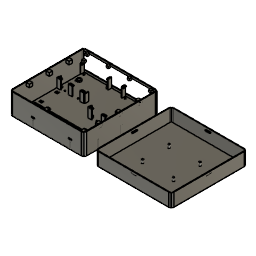
test slicing (Autodesk Fusion 360 design; units mm, degrees)
part number: 2026-06-28-20-30-48-696
Autodesk Fusion 360 part; units mm, degrees
sketch "Sketch1" plane through (0, 0, 0) normal (0, 0, 1) x (1, 0, 0)
  line L0 (140, 140) -> (-140, 140)
  line L1 (-140, 140) -> (-140, -140)
  line L2 (-140, -140) -> (140, -140)
  line L3 (140, -140) -> (140, 140)
extrude "Extrude1" add sketch "Sketch1" along normal blind 3 makes body 1
sketch "Sketch2" plane through (0, 0, 0) normal (0, 0, 1) x (1, 0, 0)
  line L0 (-137, 140) -> (-140, 140)
  line L1 (-140, 140) -> (-140, -140)
  line L2 (-140, -140) -> (-137, -140)
  line L3 (-137, -140) -> (-137, 140)
extrude "Extrude2" add sketch "Sketch2" along normal blind 77 from surface at 3 bodies 1
sketch "Sketch3" plane through (0, 0, 0) normal (0, 0, 1) x (1, 0, 0)
  line L0 (140, 140) -> (137, 140)
  line L1 (137, 140) -> (137, -140)
  line L2 (137, -140) -> (140, -140)
  line L3 (140, -140) -> (140, 140)
extrude "Extrude3" add sketch "Sketch3" along normal blind 77 from surface at 3 bodies 1
sketch "Sketch4" plane through (0, 0, 0) normal (0, 0, 1) x (1, 0, 0)
  line L0 (140, -137) -> (-140, -137)
  line L1 (-140, -137) -> (-140, -140)
  line L2 (-140, -140) -> (140, -140)
  line L3 (140, -140) -> (140, -137)
extrude "Extrude4" add sketch "Sketch4" along normal blind 77 from surface at 3 bodies 1
sketch "Sketch5" plane through (0, 0, 0) normal (0, 0, 1) x (1, 0, 0)
  line L0 (140, 140) -> (-140, 140)
  line L1 (-140, 140) -> (-140, 137)
  line L2 (-140, 137) -> (140, 137)
  line L3 (140, 137) -> (140, 140)
extrude "Extrude5" add sketch "Sketch5" along normal blind 8 from surface at 3 bodies 1
sketch "Sketch6" plane through (0, 0, 0) normal (0, 0, 1) x (1, 0, 0)
  line L0 (140, 140) -> (-140, 140)
  line L1 (-140, 140) -> (-140, 137)
  line L2 (-140, 137) -> (140, 137)
  line L3 (140, 137) -> (140, 140)
extrude "Extrude6" add sketch "Sketch6" along normal blind 8 from surface at 72 bodies 1
fillet "Fillet1" radius 10 4 edges at (-140, 140, 40) (-140, -140, 40) (140, -140, 40) (140, 140, 40) on bodies 1
sketch "Sketch7" plane through (0, 0, 0) normal (0, 0, 1) x (1, 0, 0)
  circle A0 centre (27, 128.5) radius 3.5
extrude "Extrude7" add sketch "Sketch7" along normal blind 3.5 from surface at 3 bodies 1
sketch "Sketch8" plane through (0, 0, 0) normal (0, 0, 1) x (1, 0, 0)
  circle A0 centre (27, 5.5) radius 3.5
extrude "Extrude8" add sketch "Sketch8" along normal blind 3.5 from surface at 3 bodies 1
sketch "Sketch9" plane through (0, 0, 0) normal (0, 0, 1) x (1, 0, 0)
  circle A0 centre (129, 128.5) radius 3.5
extrude "Extrude9" add sketch "Sketch9" along normal blind 3.5 from surface at 3 bodies 1
sketch "Sketch10" plane through (0, 0, 0) normal (0, 0, 1) x (1, 0, 0)
  circle A0 centre (129, 5.5) radius 3.5
extrude "Extrude10" add sketch "Sketch10" along normal blind 3.5 from surface at 3 bodies 1
sketch "Sketch11" plane through (0, 0, 0) normal (0, 0, 1) x (1, 0, 0)
  line L0 (34.5, -3) -> (20.5, -3)
  line L1 (20.5, -3) -> (20.5, -5.5)
  line L2 (20.5, -5.5) -> (34.5, -5.5)
  line L3 (34.5, -5.5) -> (34.5, -3)
extrude "Extrude11" add sketch "Sketch11" along normal blind 36.5 from surface at 3 bodies 1
sketch "Sketch12" plane through (0, 0, 0) normal (0, 0, 1) x (1, 0, 0)
  line L0 (34.5, 2.25) -> (20.5, 2.25)
  line L1 (20.5, 2.25) -> (20.5, -4.25)
  line L2 (20.5, -4.25) -> (34.5, -4.25)
  line L3 (34.5, -4.25) -> (34.5, 2.25)
extrude "Extrude12" add sketch "Sketch12" along normal blind 3 from surface at 35.5 bodies 1
sketch "Sketch13" plane through (0, 0, 0) normal (0, 0, 1) x (1, 0, 0)
  line L0 (85, -3) -> (71, -3)
  line L1 (71, -3) -> (71, -5.5)
  line L2 (71, -5.5) -> (85, -5.5)
  line L3 (85, -5.5) -> (85, -3)
extrude "Extrude13" add sketch "Sketch13" along normal blind 36.5 from surface at 3 bodies 1
sketch "Sketch14" plane through (0, 0, 0) normal (0, 0, 1) x (1, 0, 0)
  line L0 (85, 2.25) -> (71, 2.25)
  line L1 (71, 2.25) -> (71, -4.25)
  line L2 (71, -4.25) -> (85, -4.25)
  line L3 (85, -4.25) -> (85, 2.25)
extrude "Extrude14" add sketch "Sketch14" along normal blind 3 from surface at 35.5 bodies 1
sketch "Sketch15" plane through (0, 0, 0) normal (0, 0, 1) x (1, 0, 0)
  line L0 (135.5, -3) -> (121.5, -3)
  line L1 (121.5, -3) -> (121.5, -5.5)
  line L2 (121.5, -5.5) -> (135.5, -5.5)
  line L3 (135.5, -5.5) -> (135.5, -3)
extrude "Extrude15" add sketch "Sketch15" along normal blind 36.5 from surface at 3 bodies 1
sketch "Sketch16" plane through (0, 0, 0) normal (0, 0, 1) x (1, 0, 0)
  line L0 (135.5, 2.25) -> (121.5, 2.25)
  line L1 (121.5, 2.25) -> (121.5, -4.25)
  line L2 (121.5, -4.25) -> (135.5, -4.25)
  line L3 (135.5, -4.25) -> (135.5, 2.25)
extrude "Extrude16" add sketch "Sketch16" along normal blind 3 from surface at 35.5 bodies 1
sketch "Sketch17" plane through (0, 0, 0) normal (0, 0, 1) x (1, 0, 0)
  line L0 (20.5, 11) -> (18, 11)
  line L1 (18, 11) -> (18, -3)
  line L2 (18, -3) -> (20.5, -3)
  line L3 (20.5, -3) -> (20.5, 11)
extrude "Extrude17" add sketch "Sketch17" along normal blind 32.5 from surface at 3 bodies 1
sketch "Sketch18" plane through (0, 0, 0) normal (0, 0, 1) x (1, 0, 0)
  line L0 (20.5, 137) -> (18, 137)
  line L1 (18, 137) -> (18, 123)
  line L2 (18, 123) -> (20.5, 123)
  line L3 (20.5, 123) -> (20.5, 137)
extrude "Extrude18" add sketch "Sketch18" along normal blind 37.5 from surface at 3 bodies 1
sketch "Sketch19" plane through (0, 0, 0) normal (0, 0, 1) x (1, 0, 0)
  line L0 (24.5, 137) -> (18, 137)
  line L1 (18, 137) -> (18, 123)
  line L2 (18, 123) -> (24.5, 123)
  line L3 (24.5, 123) -> (24.5, 137)
extrude "Extrude19" add sketch "Sketch19" along normal blind 3 from surface at 35.5 bodies 1
sketch "Sketch20" plane through (0, 0, 0) normal (0, 0, 1) x (1, 0, 0)
  line L0 (51, 0.5) -> (48, 0.5)
  line L1 (48, 0.5) -> (48, -2.5)
  line L2 (48, -2.5) -> (51, -2.5)
  line L3 (51, -2.5) -> (51, 0.5)
extrude "Extrude20" add sketch "Sketch20" along normal blind 3 from surface at 3 bodies 1
sketch "Sketch21" plane through (0, 0, 0) normal (0, 0, 1) x (1, 0, 0)
  line L0 (138, 11) -> (135.5, 11)
  line L1 (135.5, 11) -> (135.5, -3)
  line L2 (135.5, -3) -> (138, -3)
  line L3 (138, -3) -> (138, 11)
extrude "Extrude21" add sketch "Sketch21" along normal blind 32.5 from surface at 3 bodies 1
sketch "Sketch22" plane through (0, 0, 0) normal (0, 0, 1) x (1, 0, 0)
  line L0 (138, 137) -> (135.5, 137)
  line L1 (135.5, 137) -> (135.5, 123)
  line L2 (135.5, 123) -> (138, 123)
  line L3 (138, 123) -> (138, 137)
extrude "Extrude22" add sketch "Sketch22" along normal blind 37.5 from surface at 3 bodies 1
sketch "Sketch23" plane through (0, 0, 0) normal (0, 0, 1) x (1, 0, 0)
  line L0 (138, 137) -> (131.5, 137)
  line L1 (131.5, 137) -> (131.5, 123)
  line L2 (131.5, 123) -> (138, 123)
  line L3 (138, 123) -> (138, 137)
extrude "Extrude23" add sketch "Sketch23" along normal blind 3 from surface at 35.5 bodies 1
sketch "Sketch24" plane through (0, 0, 0) normal (0, 0, 1) x (1, 0, 0)
  line L0 (108, 0.5) -> (105, 0.5)
  line L1 (105, 0.5) -> (105, -2.5)
  line L2 (105, -2.5) -> (108, -2.5)
  line L3 (108, -2.5) -> (108, 0.5)
extrude "Extrude24" add sketch "Sketch24" along normal blind 3 from surface at 3 bodies 1
sketch "Sketch25" plane through (0, 0, 0) normal (0, 0, 1) x (1, 0, 0)
  circle A0 centre (-129, 128.5) radius 3.5
extrude "Extrude25" add sketch "Sketch25" along normal blind 3.5 from surface at 3 bodies 1
sketch "Sketch26" plane through (0, 0, 0) normal (0, 0, 1) x (1, 0, 0)
  circle A0 centre (-129, 44.5) radius 3.5
extrude "Extrude26" add sketch "Sketch26" along normal blind 3.5 from surface at 3 bodies 1
sketch "Sketch27" plane through (0, 0, 0) normal (0, 0, 1) x (1, 0, 0)
  circle A0 centre (-41, 128.5) radius 3.5
extrude "Extrude27" add sketch "Sketch27" along normal blind 3.5 from surface at 3 bodies 1
sketch "Sketch28" plane through (0, 0, 0) normal (0, 0, 1) x (1, 0, 0)
  circle A0 centre (-41, 44.5) radius 3.5
extrude "Extrude28" add sketch "Sketch28" along normal blind 3.5 from surface at 3 bodies 1
sketch "Sketch29" plane through (0, 0, 0) normal (0, 0, 1) x (1, 0, 0)
  line L0 (-121.5, 36) -> (-135.5, 36)
  line L1 (-135.5, 36) -> (-135.5, 33.5)
  line L2 (-135.5, 33.5) -> (-121.5, 33.5)
  line L3 (-121.5, 33.5) -> (-121.5, 36)
extrude "Extrude29" add sketch "Sketch29" along normal blind 35.5 from surface at 3 bodies 1
sketch "Sketch30" plane through (0, 0, 0) normal (0, 0, 1) x (1, 0, 0)
  line L0 (-121.5, 41.25) -> (-135.5, 41.25)
  line L1 (-135.5, 41.25) -> (-135.5, 34.75)
  line L2 (-135.5, 34.75) -> (-121.5, 34.75)
  line L3 (-121.5, 34.75) -> (-121.5, 41.25)
extrude "Extrude30" add sketch "Sketch30" along normal blind 3 from surface at 34.5 bodies 1
sketch "Sketch31" plane through (0, 0, 0) normal (0, 0, 1) x (1, 0, 0)
  line L0 (-78, 36) -> (-92, 36)
  line L1 (-92, 36) -> (-92, 33.5)
  line L2 (-92, 33.5) -> (-78, 33.5)
  line L3 (-78, 33.5) -> (-78, 36)
extrude "Extrude31" add sketch "Sketch31" along normal blind 35.5 from surface at 3 bodies 1
sketch "Sketch32" plane through (0, 0, 0) normal (0, 0, 1) x (1, 0, 0)
  line L0 (-78, 41.25) -> (-92, 41.25)
  line L1 (-92, 41.25) -> (-92, 34.75)
  line L2 (-92, 34.75) -> (-78, 34.75)
  line L3 (-78, 34.75) -> (-78, 41.25)
extrude "Extrude32" add sketch "Sketch32" along normal blind 3 from surface at 34.5 bodies 1
sketch "Sketch33" plane through (0, 0, 0) normal (0, 0, 1) x (1, 0, 0)
  line L0 (-34.5, 36) -> (-48.5, 36)
  line L1 (-48.5, 36) -> (-48.5, 33.5)
  line L2 (-48.5, 33.5) -> (-34.5, 33.5)
  line L3 (-34.5, 33.5) -> (-34.5, 36)
extrude "Extrude33" add sketch "Sketch33" along normal blind 35.5 from surface at 3 bodies 1
sketch "Sketch34" plane through (0, 0, 0) normal (0, 0, 1) x (1, 0, 0)
  line L0 (-34.5, 41.25) -> (-48.5, 41.25)
  line L1 (-48.5, 41.25) -> (-48.5, 34.75)
  line L2 (-48.5, 34.75) -> (-34.5, 34.75)
  line L3 (-34.5, 34.75) -> (-34.5, 41.25)
extrude "Extrude34" add sketch "Sketch34" along normal blind 3 from surface at 34.5 bodies 1
sketch "Sketch35" plane through (0, 0, 0) normal (0, 0, 1) x (1, 0, 0)
  line L0 (-135.5, 50) -> (-138, 50)
  line L1 (-138, 50) -> (-138, 36)
  line L2 (-138, 36) -> (-135.5, 36)
  line L3 (-135.5, 36) -> (-135.5, 50)
extrude "Extrude35" add sketch "Sketch35" along normal blind 31.5 from surface at 3 bodies 1
sketch "Sketch36" plane through (0, 0, 0) normal (0, 0, 1) x (1, 0, 0)
  line L0 (-135.5, 137) -> (-138, 137)
  line L1 (-138, 137) -> (-138, 123)
  line L2 (-138, 123) -> (-135.5, 123)
  line L3 (-135.5, 123) -> (-135.5, 137)
extrude "Extrude36" add sketch "Sketch36" along normal blind 36.5 from surface at 3 bodies 1
sketch "Sketch37" plane through (0, 0, 0) normal (0, 0, 1) x (1, 0, 0)
  line L0 (-131.5, 137) -> (-138, 137)
  line L1 (-138, 137) -> (-138, 123)
  line L2 (-138, 123) -> (-131.5, 123)
  line L3 (-131.5, 123) -> (-131.5, 137)
extrude "Extrude37" add sketch "Sketch37" along normal blind 3 from surface at 34.5 bodies 1
sketch "Sketch38" plane through (0, 0, 0) normal (0, 0, 1) x (1, 0, 0)
  line L0 (-108.5, 39.5) -> (-111.5, 39.5)
  line L1 (-111.5, 39.5) -> (-111.5, 36.5)
  line L2 (-111.5, 36.5) -> (-108.5, 36.5)
  line L3 (-108.5, 36.5) -> (-108.5, 39.5)
extrude "Extrude38" add sketch "Sketch38" along normal blind 3 from surface at 3 bodies 1
sketch "Sketch39" plane through (0, 0, 0) normal (0, 0, 1) x (1, 0, 0)
  line L0 (-32, 50) -> (-34.5, 50)
  line L1 (-34.5, 50) -> (-34.5, 36)
  line L2 (-34.5, 36) -> (-32, 36)
  line L3 (-32, 36) -> (-32, 50)
extrude "Extrude39" add sketch "Sketch39" along normal blind 31.5 from surface at 3 bodies 1
sketch "Sketch40" plane through (0, 0, 0) normal (0, 0, 1) x (1, 0, 0)
  line L0 (-32, 137) -> (-34.5, 137)
  line L1 (-34.5, 137) -> (-34.5, 123)
  line L2 (-34.5, 123) -> (-32, 123)
  line L3 (-32, 123) -> (-32, 137)
extrude "Extrude40" add sketch "Sketch40" along normal blind 36.5 from surface at 3 bodies 1
sketch "Sketch41" plane through (0, 0, 0) normal (0, 0, 1) x (1, 0, 0)
  line L0 (-32, 137) -> (-38.5, 137)
  line L1 (-38.5, 137) -> (-38.5, 123)
  line L2 (-38.5, 123) -> (-32, 123)
  line L3 (-32, 123) -> (-32, 137)
extrude "Extrude41" add sketch "Sketch41" along normal blind 3 from surface at 34.5 bodies 1
sketch "Sketch42" plane through (0, 0, 0) normal (0, 0, 1) x (1, 0, 0)
  line L0 (-58.5, 39.5) -> (-61.5, 39.5)
  line L1 (-61.5, 39.5) -> (-61.5, 36.5)
  line L2 (-61.5, 36.5) -> (-58.5, 36.5)
  line L3 (-58.5, 36.5) -> (-58.5, 39.5)
extrude "Extrude42" add sketch "Sketch42" along normal blind 3 from surface at 3 bodies 1
sketch "Sketch43" plane through (0, 0, 0) normal (0, 0, 1) x (1, 0, 0)
  line L0 (137, -83.5) -> (-103, -83.5)
  line L1 (-103, -83.5) -> (-103, -86.5)
  line L2 (-103, -86.5) -> (137, -86.5)
  line L3 (137, -86.5) -> (137, -83.5)
extrude "Extrude43" add sketch "Sketch43" along normal blind 29 from surface at 3 bodies 1
sketch "Sketch44" plane through (0, 0, 0) normal (0, 0, 1) x (1, 0, 0)
  circle A0 centre (-53, -83) radius 3
extrude "Extrude44" add sketch "Sketch44" along normal blind 29 from surface at 3 bodies 1
sketch "Sketch45" plane through (0, 0, 0) normal (0, 0, 1) x (1, 0, 0)
  circle A0 centre (-53, -83) radius 1.3
extrude "Extrude45" cut sketch "Sketch45" along normal blind 11 from surface at 23 bodies 1
sketch "Sketch46" plane through (0, 0, 0) normal (0, 0, 1) x (1, 0, 0)
  circle A0 centre (-53, -136.5) radius 3
extrude "Extrude46" add sketch "Sketch46" along normal blind 29 from surface at 3 bodies 1
sketch "Sketch47" plane through (0, 0, 0) normal (0, 0, 1) x (1, 0, 0)
  circle A0 centre (-53, -136.5) radius 1.3
extrude "Extrude47" cut sketch "Sketch47" along normal blind 11 from surface at 23 bodies 1
sketch "Sketch48" plane through (0, 0, 0) normal (0, 0, 1) x (1, 0, 0)
  line L0 (-47, -79) -> (-59, -79)
  line L1 (-59, -79) -> (-59, -139.5)
  line L2 (-59, -139.5) -> (-47, -139.5)
  line L3 (-47, -139.5) -> (-47, -79)
extrude "Extrude48" add sketch "Sketch48" along normal blind 4 from surface at 32 separate body makes body 2
sketch "Sketch49" plane through (0, 0, 0) normal (0, 0, 1) x (1, 0, 0)
  circle A0 centre (-53, -83) radius 1.8
extrude "Extrude49" cut sketch "Sketch49" along normal blind 6 from surface at 31 bodies 2
sketch "Sketch50" plane through (0, 0, 0) normal (0, 0, 1) x (1, 0, 0)
  circle A0 centre (-53, -136.5) radius 1.8
extrude "Extrude50" cut sketch "Sketch50" along normal blind 6 from surface at 31 bodies 2
sketch "Sketch51" plane through (0, 0, 0) normal (0, 0, 1) x (1, 0, 0)
  circle A0 centre (87, -83) radius 3
extrude "Extrude51" add sketch "Sketch51" along normal blind 29 from surface at 3 bodies 1
sketch "Sketch52" plane through (0, 0, 0) normal (0, 0, 1) x (1, 0, 0)
  circle A0 centre (87, -83) radius 1.3
extrude "Extrude52" cut sketch "Sketch52" along normal blind 11 from surface at 23 bodies 1
sketch "Sketch53" plane through (0, 0, 0) normal (0, 0, 1) x (1, 0, 0)
  circle A0 centre (87, -136.5) radius 3
extrude "Extrude53" add sketch "Sketch53" along normal blind 29 from surface at 3 bodies 1
sketch "Sketch54" plane through (0, 0, 0) normal (0, 0, 1) x (1, 0, 0)
  circle A0 centre (87, -136.5) radius 1.3
extrude "Extrude54" cut sketch "Sketch54" along normal blind 11 from surface at 23 bodies 1
sketch "Sketch55" plane through (0, 0, 0) normal (0, 0, 1) x (1, 0, 0)
  line L0 (93, -79) -> (81, -79)
  line L1 (81, -79) -> (81, -139.5)
  line L2 (81, -139.5) -> (93, -139.5)
  line L3 (93, -139.5) -> (93, -79)
extrude "Extrude55" add sketch "Sketch55" along normal blind 4 from surface at 32 separate body makes body 3
sketch "Sketch56" plane through (0, 0, 0) normal (0, 0, 1) x (1, 0, 0)
  circle A0 centre (87, -83) radius 1.8
extrude "Extrude56" cut sketch "Sketch56" along normal blind 6 from surface at 31 bodies 3
sketch "Sketch57" plane through (0, 0, 0) normal (0, 0, 1) x (1, 0, 0)
  circle A0 centre (87, -136.5) radius 1.8
extrude "Extrude57" cut sketch "Sketch57" along normal blind 6 from surface at 31 bodies 3
sketch "Sketch58" plane through (0, 0, 0) normal (0, 0, 1) x (1, 0, 0)
  circle A0 centre (-118, 100) radius 5
extrude "Extrude58" cut sketch "Sketch58" along normal blind 5 from surface at -1 bodies 1
sketch "Sketch59" plane through (0, 0, 0) normal (0, 0, 1) x (1, 0, 0)
  circle A0 centre (-118, 100) radius 8
extrude "Extrude59" add sketch "Sketch59" along normal blind 4 from surface at 3 bodies 1
sketch "Sketch60" plane through (0, 0, 0) normal (0, 0, 1) x (1, 0, 0)
  circle A0 centre (-118, 100) radius 5
extrude "Extrude60" cut sketch "Sketch60" along normal blind 6 from surface at 2 bodies 1
sketch "Sketch61" plane through (0, 0, 0) normal (0, 0, 1) x (1, 0, 0)
  line L0 (-116, -65.5) -> (-120, -65.5)
  line L1 (-120, -65.5) -> (-120, -74.5)
  line L2 (-120, -74.5) -> (-116, -74.5)
  line L3 (-116, -74.5) -> (-116, -65.5)
extrude "Extrude61" cut sketch "Sketch61" along normal blind 5 from surface at -1 bodies 1
sketch "Sketch62" plane through (0, 0, 0) normal (0, 0, 1) x (1, 0, 0)
  line L0 (-122, -65.5) -> (-126, -65.5)
  line L1 (-126, -65.5) -> (-126, -74.5)
  line L2 (-126, -74.5) -> (-122, -74.5)
  line L3 (-122, -74.5) -> (-122, -65.5)
extrude "Extrude62" cut sketch "Sketch62" along normal blind 5 from surface at -1 bodies 1
sketch "Sketch63" plane through (0, 0, 0) normal (0, 0, 1) x (1, 0, 0)
  line L0 (-116, -35.5) -> (-120, -35.5)
  line L1 (-120, -35.5) -> (-120, -44.5)
  line L2 (-120, -44.5) -> (-116, -44.5)
  line L3 (-116, -44.5) -> (-116, -35.5)
extrude "Extrude63" cut sketch "Sketch63" along normal blind 5 from surface at -1 bodies 1
sketch "Sketch64" plane through (0, 0, 0) normal (0, 0, 1) x (1, 0, 0)
  line L0 (-122, -35.5) -> (-126, -35.5)
  line L1 (-126, -35.5) -> (-126, -44.5)
  line L2 (-126, -44.5) -> (-122, -44.5)
  line L3 (-122, -44.5) -> (-122, -35.5)
extrude "Extrude64" cut sketch "Sketch64" along normal blind 5 from surface at -1 bodies 1
sketch "Sketch65" plane through (0, 0, 0) normal (0, 0, 1) x (1, 0, 0)
  line L0 (-116, 24.5) -> (-120, 24.5)
  line L1 (-120, 24.5) -> (-120, 15.5)
  line L2 (-120, 15.5) -> (-116, 15.5)
  line L3 (-116, 15.5) -> (-116, 24.5)
extrude "Extrude65" cut sketch "Sketch65" along normal blind 5 from surface at -1 bodies 1
sketch "Sketch66" plane through (0, 0, 0) normal (0, 0, 1) x (1, 0, 0)
  line L0 (-122, 24.5) -> (-126, 24.5)
  line L1 (-126, 24.5) -> (-126, 15.5)
  line L2 (-126, 15.5) -> (-122, 15.5)
  line L3 (-122, 15.5) -> (-122, 24.5)
extrude "Extrude66" cut sketch "Sketch66" along normal blind 5 from surface at -1 bodies 1
sketch "Sketch67" plane through (0, 0, 0) normal (0, 0, 1) x (1, 0, 0)
  line L0 (-116, 101) -> (-120, 101)
  line L1 (-120, 101) -> (-120, 92)
  line L2 (-120, 92) -> (-116, 92)
  line L3 (-116, 92) -> (-116, 101)
extrude "Extrude67" cut sketch "Sketch67" along normal blind 5 from surface at -1 bodies 1
sketch "Sketch68" plane through (0, 0, 0) normal (0, 0, 1) x (1, 0, 0)
  line L0 (-122, 101) -> (-126, 101)
  line L1 (-126, 101) -> (-126, 92)
  line L2 (-126, 92) -> (-122, 92)
  line L3 (-122, 92) -> (-122, 101)
extrude "Extrude68" cut sketch "Sketch68" along normal blind 5 from surface at -1 bodies 1
sketch "Sketch69" plane through (0, 0, 0) normal (0, 1, 0) x (1, 0, 0)
  circle A0 centre (-60, 56) radius 5.5
extrude "Extrude69" cut sketch "Sketch69" along normal mid plane 5 from surface at -139 bodies 1
sketch "Sketch70" plane through (0, 0, 0) normal (0, 1, 0) x (1, 0, 0)
  line L0 (-57.5, 56) -> (-62.5, 56)
  line L1 (-62.5, 56) -> (-62.5, 38)
  line L2 (-62.5, 38) -> (-57.5, 38)
  line L3 (-57.5, 38) -> (-57.5, 56)
extrude "Extrude70" cut sketch "Sketch70" along normal mid plane 5 from surface at -139 bodies 1
sketch "Sketch71" plane through (0, 0, 0) normal (0, 1, 0) x (1, 0, 0)
  circle A0 centre (60, 56) radius 5.5
extrude "Extrude71" cut sketch "Sketch71" along normal mid plane 5 from surface at -139 bodies 1
sketch "Sketch72" plane through (0, 0, 0) normal (0, 1, 0) x (1, 0, 0)
  line L0 (62.5, 56) -> (57.5, 56)
  line L1 (57.5, 56) -> (57.5, 38)
  line L2 (57.5, 38) -> (62.5, 38)
  line L3 (62.5, 38) -> (62.5, 56)
extrude "Extrude72" cut sketch "Sketch72" along normal mid plane 5 from surface at -139 bodies 1
sketch "Sketch73" plane through (0, 0, 0) normal (0, 0, 1) x (1, 0, 0)
  line L0 (-125, -69) -> (-137, -69)
  line L1 (-137, -69) -> (-137, -81)
  line L2 (-137, -81) -> (-125, -81)
  line L3 (-125, -81) -> (-125, -69)
extrude "Extrude73" add sketch "Sketch73" along normal blind 12 from surface at 66 bodies 1
sketch "Sketch74" plane through (0, 0, 0) normal (1, 0, 0) x (0, 0, -1)
  circle A0 centre (-75, 72) radius 1.3
extrude "Extrude74" cut sketch "Sketch74" along normal mid plane 30 from surface at -137 bodies 1
sketch "Sketch75" plane through (0, 0, 0) normal (0, 0, 1) x (1, 0, 0)
  line L0 (-125, 6) -> (-137, 6)
  line L1 (-137, 6) -> (-137, -6)
  line L2 (-137, -6) -> (-125, -6)
  line L3 (-125, -6) -> (-125, 6)
extrude "Extrude75" add sketch "Sketch75" along normal blind 12 from surface at 66 bodies 1
sketch "Sketch76" plane through (0, 0, 0) normal (1, 0, 0) x (0, 0, -1)
  circle A0 centre (0, 72) radius 1.3
extrude "Extrude76" cut sketch "Sketch76" along normal mid plane 30 from surface at -137 bodies 1
sketch "Sketch77" plane through (0, 0, 0) normal (0, 0, 1) x (1, 0, 0)
  line L0 (-125, 81) -> (-137, 81)
  line L1 (-137, 81) -> (-137, 69)
  line L2 (-137, 69) -> (-125, 69)
  line L3 (-125, 69) -> (-125, 81)
extrude "Extrude77" add sketch "Sketch77" along normal blind 12 from surface at 66 bodies 1
sketch "Sketch78" plane through (0, 0, 0) normal (1, 0, 0) x (0, 0, -1)
  circle A0 centre (75, 72) radius 1.3
extrude "Extrude78" cut sketch "Sketch78" along normal mid plane 30 from surface at -137 bodies 1
sketch "Sketch79" plane through (0, 0, 0) normal (0, 0, 1) x (1, 0, 0)
  line L0 (137, -69) -> (125, -69)
  line L1 (125, -69) -> (125, -81)
  line L2 (125, -81) -> (137, -81)
  line L3 (137, -81) -> (137, -69)
extrude "Extrude79" add sketch "Sketch79" along normal blind 12 from surface at 66 bodies 1
sketch "Sketch80" plane through (0, 0, 0) normal (1, 0, 0) x (0, 0, -1)
  circle A0 centre (-75, 72) radius 1.3
extrude "Extrude80" cut sketch "Sketch80" along normal mid plane 30 from surface at 137 bodies 1
sketch "Sketch81" plane through (0, 0, 0) normal (0, 0, 1) x (1, 0, 0)
  line L0 (137, 6) -> (125, 6)
  line L1 (125, 6) -> (125, -6)
  line L2 (125, -6) -> (137, -6)
  line L3 (137, -6) -> (137, 6)
extrude "Extrude81" add sketch "Sketch81" along normal blind 12 from surface at 66 bodies 1
sketch "Sketch82" plane through (0, 0, 0) normal (1, 0, 0) x (0, 0, -1)
  circle A0 centre (0, 72) radius 1.3
extrude "Extrude82" cut sketch "Sketch82" along normal mid plane 30 from surface at 137 bodies 1
sketch "Sketch83" plane through (0, 0, 0) normal (0, 0, 1) x (1, 0, 0)
  line L0 (137, 81) -> (125, 81)
  line L1 (125, 81) -> (125, 69)
  line L2 (125, 69) -> (137, 69)
  line L3 (137, 69) -> (137, 81)
extrude "Extrude83" add sketch "Sketch83" along normal blind 12 from surface at 66 bodies 1
sketch "Sketch84" plane through (0, 0, 0) normal (1, 0, 0) x (0, 0, -1)
  circle A0 centre (75, 72) radius 1.3
extrude "Extrude84" cut sketch "Sketch84" along normal mid plane 30 from surface at 137 bodies 1
sketch "Sketch85" plane through (0, 0, 0) normal (0, 0, 1) x (1, 0, 0)
  line L0 (-137, 137) -> (-140, 137)
  line L1 (-140, 137) -> (-140, 134)
  line L2 (-140, 134) -> (-137, 134)
  line L3 (-137, 134) -> (-137, 137)
extrude "Extrude85" add sketch "Sketch85" along normal blind 77 from surface at 3 bodies 1
sketch "Sketch86" plane through (0, 0, 0) normal (0, 0, 1) x (1, 0, 0)
  line L0 (140, 137) -> (137, 137)
  line L1 (137, 137) -> (137, 134)
  line L2 (137, 134) -> (140, 134)
  line L3 (140, 134) -> (140, 137)
extrude "Extrude86" add sketch "Sketch86" along normal blind 77 from surface at 3 bodies 1
sketch "Sketch87" plane through (0, 0, 0) normal (0, 0, 1) x (1, 0, 0)
  line L0 (-115.5, 137) -> (-124.5, 137)
  line L1 (-124.5, 137) -> (-124.5, 128)
  line L2 (-124.5, 128) -> (-115.5, 128)
  line L3 (-115.5, 128) -> (-115.5, 137)
extrude "Extrude87" add sketch "Sketch87" along normal blind 8 from surface at 68 bodies 1
sketch "Sketch88" plane through (0, 0, 0) normal (0, 1, 0) x (1, 0, 0)
  circle A0 centre (-120, 72) radius 1.3
extrude "Extrude88" cut sketch "Sketch88" along normal mid plane 16 from surface at 132.5 bodies 1
sketch "Sketch89" plane through (0, 0, 0) normal (0, 0, 1) x (1, 0, 0)
  line L0 (124.5, 137) -> (115.5, 137)
  line L1 (115.5, 137) -> (115.5, 128)
  line L2 (115.5, 128) -> (124.5, 128)
  line L3 (124.5, 128) -> (124.5, 137)
extrude "Extrude89" add sketch "Sketch89" along normal blind 8 from surface at 68 bodies 1
sketch "Sketch90" plane through (0, 0, 0) normal (0, 1, 0) x (1, 0, 0)
  circle A0 centre (120, 72) radius 1.3
extrude "Extrude90" cut sketch "Sketch90" along normal mid plane 16 from surface at 132.5 bodies 1
sketch "Sketch91" plane through (0, 0, 0) normal (0, 0, 1) x (1, 0, 0)
  line L0 (-35.5, 137) -> (-44.5, 137)
  line L1 (-44.5, 137) -> (-44.5, 128)
  line L2 (-44.5, 128) -> (-35.5, 128)
  line L3 (-35.5, 128) -> (-35.5, 137)
extrude "Extrude91" add sketch "Sketch91" along normal blind 8 from surface at 68 bodies 1
sketch "Sketch92" plane through (0, 0, 0) normal (0, 1, 0) x (1, 0, 0)
  circle A0 centre (-40, 72) radius 1.3
extrude "Extrude92" cut sketch "Sketch92" along normal mid plane 16 from surface at 132.5 bodies 1
sketch "Sketch93" plane through (0, 0, 0) normal (0, 0, 1) x (1, 0, 0)
  line L0 (44.5, 137) -> (35.5, 137)
  line L1 (35.5, 137) -> (35.5, 128)
  line L2 (35.5, 128) -> (44.5, 128)
  line L3 (44.5, 128) -> (44.5, 137)
extrude "Extrude93" add sketch "Sketch93" along normal blind 8 from surface at 68 bodies 1
sketch "Sketch94" plane through (0, 0, 0) normal (0, 1, 0) x (1, 0, 0)
  circle A0 centre (40, 72) radius 1.3
extrude "Extrude94" cut sketch "Sketch94" along normal mid plane 16 from surface at 132.5 bodies 1
sketch "Sketch95" plane through (0, 0, 0) normal (0, 0, 1) x (1, 0, 0)
  line L0 (-127.5, 137) -> (-136.5, 137)
  line L1 (-136.5, 137) -> (-136.5, 128)
  line L2 (-136.5, 128) -> (-127.5, 128)
  line L3 (-127.5, 128) -> (-127.5, 137)
extrude "Extrude95" add sketch "Sketch95" along normal blind 8 from surface at 40 bodies 1 makes body 4
sketch "Sketch96" plane through (0, 0, 0) normal (0, 1, 0) x (1, 0, 0)
  circle A0 centre (-132, 44) radius 1.3
extrude "Extrude96" cut sketch "Sketch96" along normal mid plane 16 from surface at 132.5 bodies 1
sketch "Sketch97" plane through (0, 0, 0) normal (0, 0, 1) x (1, 0, 0)
  line L0 (136.5, 137) -> (127.5, 137)
  line L1 (127.5, 137) -> (127.5, 128)
  line L2 (127.5, 128) -> (136.5, 128)
  line L3 (136.5, 128) -> (136.5, 137)
extrude "Extrude97" add sketch "Sketch97" along normal blind 8 from surface at 40 bodies 1
sketch "Sketch98" plane through (0, 0, 0) normal (0, 1, 0) x (1, 0, 0)
  circle A0 centre (132, 44) radius 1.3
extrude "Extrude98" cut sketch "Sketch98" along normal mid plane 16 from surface at 132.5 bodies 1
sketch "Sketch99" plane through (0, 0, 0) normal (0, 0, 1) x (1, 0, 0)
  line L0 (473, 143) -> (187, 143)
  line L1 (187, 143) -> (187, -143)
  line L2 (187, -143) -> (473, -143)
  line L3 (473, -143) -> (473, 143)
extrude "Extrude99" add sketch "Sketch99" along normal blind 3 separate body makes body 5
sketch "Sketch100" plane through (0, 0, 0) normal (0, 0, 1) x (1, 0, 0)
  line L0 (473, 143) -> (187, 143)
  line L1 (187, 143) -> (187, -143)
  line L2 (187, -143) -> (473, -143)
  line L3 (473, -143) -> (473, 143)
extrude "Extrude100" add sketch "Sketch100" along normal blind 47 from surface at 3 bodies 5
sketch "Sketch101" plane through (0, 0, 0) normal (0, 0, 1) x (1, 0, 0)
  line L0 (470.5, 140.5) -> (189.5, 140.5)
  line L1 (189.5, 140.5) -> (189.5, -140.5)
  line L2 (189.5, -140.5) -> (470.5, -140.5)
  line L3 (470.5, -140.5) -> (470.5, 140.5)
extrude "Extrude101" cut sketch "Sketch101" along normal blind 49 from surface at 2 bodies 5
fillet "Fillet2" radius 10 4 edges at (473, -143, 25) (187, -143, 25) (187, 143, 25) (473, 143, 25) on bodies 5
sketch "Sketch102" plane through (0, 0, 0) normal (0, 0, 1) x (1, 0, 0)
  circle A0 centre (271.5, -50) radius 3.5
extrude "Extrude102" add sketch "Sketch102" along normal blind 12 from surface at 3 bodies 5 makes body 6
sketch "Sketch103" plane through (0, 0, 0) normal (0, 0, 1) x (1, 0, 0)
  circle A0 centre (271.5, -50) radius 1.3
extrude "Extrude103" cut sketch "Sketch103" along normal blind 13 from surface at 3 bodies 5
sketch "Sketch104" plane through (0, 0, 0) normal (0, 0, 1) x (1, 0, 0)
  circle A0 centre (271.5, 50) radius 3.5
extrude "Extrude104" add sketch "Sketch104" along normal blind 12 from surface at 3 bodies 5 makes body 7
sketch "Sketch105" plane through (0, 0, 0) normal (0, 0, 1) x (1, 0, 0)
  circle A0 centre (271.5, 50) radius 1.3
extrude "Extrude105" cut sketch "Sketch105" along normal blind 13 from surface at 3 bodies 5
sketch "Sketch106" plane through (0, 0, 0) normal (0, 0, 1) x (1, 0, 0)
  circle A0 centre (388.5, -50) radius 3.5
extrude "Extrude106" add sketch "Sketch106" along normal blind 12 from surface at 3 bodies 5 makes body 8
sketch "Sketch107" plane through (0, 0, 0) normal (0, 0, 1) x (1, 0, 0)
  circle A0 centre (388.5, -50) radius 1.3
extrude "Extrude107" cut sketch "Sketch107" along normal blind 13 from surface at 3 bodies 5
sketch "Sketch108" plane through (0, 0, 0) normal (0, 0, 1) x (1, 0, 0)
  circle A0 centre (388.5, 50) radius 3.5
extrude "Extrude108" add sketch "Sketch108" along normal blind 12 from surface at 3 bodies 5 makes body 9
sketch "Sketch109" plane through (0, 0, 0) normal (0, 0, 1) x (1, 0, 0)
  circle A0 centre (388.5, 50) radius 1.3
extrude "Extrude109" cut sketch "Sketch109" along normal blind 13 from surface at 3 bodies 5
sketch "Sketch110" plane through (0, 0, 0) normal (0, 0, 1) x (1, 0, 0)
  line L0 (472.5, 10) -> (466.5, 10)
  line L1 (466.5, 10) -> (466.5, -10)
  line L2 (466.5, -10) -> (472.5, -10)
  line L3 (472.5, -10) -> (472.5, 10)
extrude "Extrude110" add sketch "Sketch110" along normal blind 2 from surface at 40 bodies 5
sketch "Sketch111" plane through (0, 0, 0) normal (0, 0, 1) x (1, 0, 0)
  line L0 (193.5, 10) -> (187.5, 10)
  line L1 (187.5, 10) -> (187.5, -10)
  line L2 (187.5, -10) -> (193.5, -10)
  line L3 (193.5, -10) -> (193.5, 10)
extrude "Extrude111" add sketch "Sketch111" along normal blind 2 from surface at 40 bodies 5
sketch "Sketch112" plane through (0, 0, 0) normal (0, 0, 1) x (1, 0, 0)
  line L0 (340, 142.5) -> (320, 142.5)
  line L1 (320, 142.5) -> (320, 136.5)
  line L2 (320, 136.5) -> (340, 136.5)
  line L3 (340, 136.5) -> (340, 142.5)
extrude "Extrude112" add sketch "Sketch112" along normal blind 2 from surface at 40 bodies 5
sketch "Sketch113" plane through (0, 0, 0) normal (0, 0, 1) x (1, 0, 0)
  line L0 (340, -136.5) -> (320, -136.5)
  line L1 (320, -136.5) -> (320, -142.5)
  line L2 (320, -142.5) -> (340, -142.5)
  line L3 (340, -142.5) -> (340, -136.5)
extrude "Extrude113" add sketch "Sketch113" along normal blind 2 from surface at 40 bodies 5
named bodies: "FIR SHELL (tub)", "FIR EXT STRAP (screws down)", "FIR EXT STRAP (screws down) (1)", "FIR TOP LID (deep cap)"
